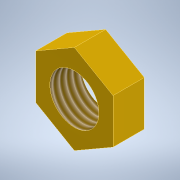
# Autodesk Inventor part: mutter
Saved by Autodesk Inventor 2021 (Build 250183000, 183)
## iProperties
Created: 2021-02-09
Part Number: mutter
Material: Generic
Document SubType Name: Modeling
Designer: Emil
Density: 1 g/cm^3
Appearance: Gold
Author: Emil
Autodesk Inventor part; units mm, degrees
ref_plane "YZ Plane" through (0, 0, 0) normal (1, 0, 0) x (0, 1, 0)
ref_plane "XZ Plane" through (0, 0, 0) normal (0, 1, 0) x (-1, 0, 0)
ref_plane "XY Plane" through (0, 0, 0) normal (0, 0, 1) x (1, 0, 0)
sketch "Sketch1" plane through (0, 0, 0) normal (0, 0, 1) x (1, 0, 0)
  line L0 (0, 12.846) -> (0, -12.1789)
  line L1 (0, 8.6963) -> (-8.6603, 3.6963)
  line L2 (-8.6603, 3.6963) -> (-8.6603, -6.3037)
  line L3 (-8.6603, -6.3037) -> (0, -11.3037)
  line L4 (0, 8.6963) -> (8.6603, 3.6963)
  line L5 (8.6603, 3.6963) -> (8.6603, -6.3037)
  line L6 (8.6603, -6.3037) -> (0, -11.3037)
  point P0 (0, 0)
  dimension "d0" = 120
  dimension "d1" = 120
  dimension "d2" = 10
  dimension "d4" = 5
  dimension "d16" = 9.7893
  dimension "d17" = 20.9142
  dimension "d18" = 0.758
  constraints: 14 end point, 3 point on line, 2 symmetric about line, 2 vertical
  measures "d0" angle of L2 L1
  measures "d1" angle of L3 L2
  measures "d2" distance of L1.end L2.end
  measures "d4" vertical distance of L1.start L1.end
  measures "d16" distance from line of point (0, 0) L6
  measures "d17" distance from line of L0.start L6
  measures "d18" distance from line of L0.end L6
extrude "Extrusion1" add sketch "Sketch1" along normal blind 7
sketch "Sketch2" plane through (0, 0, 7) normal (0, 0, 1) x (1, 0, 0)
  line L0 (0, 10.2692) -> (0, -14.045)
  line L1 (8.6603, -6.3037) -> (8.6603, 3.6963) projected
  line L2 (8.6603, -1.3037) -> (-8.6603, -1.3037)
  line L3 (-8.6603, 3.6963) -> (-8.6603, -6.3037) projected
  point P0 (0, 0)
  point P1 (0, -1.3037)
  dimension "d22" = 8.6602
  dimension "d23" = 23.1456
  dimension "d24" = 25.4826
  constraints: 4 end point, 3 midpoint, 1 vertical
  measures "d22" distance between parallel lines of L0 L1
  measures "d23" diameter of L0.start L2
  measures "d24" diameter of L0.end L2
hole "Hole1" at (0, -1.3037, 7) direction (0, 0, -1) diameter 11 end through all
thread "Thread2" size "M11x1.5" class "6H" standard "ANSI Metric M Profile" full length
equation "\"d4\" = 0.5 * d2"
body "Solid1"
